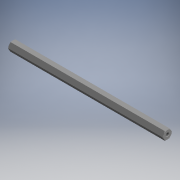
# Autodesk Inventor part: SLSBF7-130-M3-N3
Saved by Autodesk Inventor 2017.3 (Build 213256000, 256)
## iProperties
Part Number: SLSBF7-130-M3-N3
Material: Generic
Catalog Web Link: www.cadenas.de
Description: NLSBF, LSBF, PLSBF, BLSBF, SLSBF, ALSBF, ABLSBF-Hex Posts - Both Ends Tapped - L Dimension, Thread Dia. Configurable -
Vendor: MISUMI
Document SubType Name: Modeling
Designer: partserver
Manufacturer: MISUMI
Mass: 5.43424 g
Surface Area: 33.6052 cm^2
Volume: 5.43424 cm^3
Density: 1 g/cm^3
Appearance: PSOLRGB-175-175-175
Category: PARTsolutions
Company: MISUMI
Title: SLSBF7-130-M3-N3
Author: Cadenas PARTsolutions
Comments: Hex Posts - Both Ends Tapped - L Dimension, Thread Dia. Configurable -
PSOL_IDENT_0: {$CADENAS_DATA\23d-libs\misumi\metric\19_posts_stands\plsbf.prj},250 {VTYP=3D},{NB=SLSBF7-130-M3-N3}
PSOL_IDENT_1: ,{LINA=SLSBF7-130-M3-N3},{NN=NLSBF, LSBF, PLSBF, BLSBF, SLSBF, ALSBF, ABLSBF},{DATE=02.06.2021 23:49
PSOL_IDENT_2: :08},{GEOMDATE=25.03.2021 00:56:23},{VERSION=},{LINEID=50},{WBVAR=MAT,ST,M,N,ALT1,L,ALT4,ALT2,ALT3},
PSOL_IDENT_3: {WBNUMERIC=M,N,L}  {NB=SLSBF7-130-M3-N3},{LINA=SLSBF7-130-M3-N3},{KT=DUMMY},{PN=SLSBF7-130-M3-N3},{T
PSOL_IDENT_4: YPE=SLSBF},{MAT=304},{MATALG= 'LCS','Low Carbon Steel','304','SUS304','A2011','A2011 Aluminum Alloy'
PSOL_IDENT_5: },{ST=-},{STALG= '-','-' },{B=7},{M=3},{MALG=[3,4,5]},{N=3},{NALG=[3,4,5]},{ALT1=},{L=130.0},{LALG=
PSOL_IDENT_6: [15:200/0.5]},{LMIN=15},{LMIN1=12},{LMIN1ALG=12},{LMIN2=15.000},{C=8.1},{ALT4=},{ALT4ALG= '', 'w/o L
PSOL_IDENT_7: VC (L Dimension Accuracy Change)', 'LVC', 'with LVC (L Dimension Accuracy Change)'},{ALT4PN=},{ALT2=
PSOL_IDENT_8: },{ALT2ALG='','w/o MD (Left End Change The Effective Tap Depth)','MD','with MD (Left End Change The
PSOL_IDENT_9: Effective Tap Depth)'},{ALT2PN=},{ALT3=},{ALT3ALG='','w/o ND (Right End Change The Effective Tap Dep
PSOL_IDENT_10: th)','ND','with ND (Right End Change The Effective Tap Depth)'},{ALT3PN=},{MAV=3},{MPITCH=0.5},{NPIT
PSOL_IDENT_11: CH=0.5},{NDEPT=9},{MDEPT=9},{M3D=6},{N3D=6}
NB: SLSBF7-130-M3-N3
NN: NLSBF, LSBF, PLSBF, BLSBF, SLSBF, ALSBF, ABLSBF
NT: Hex Posts - Both Ends Tapped - L Dimension, Thread Dia. Configurable -
NBSYN: $PN.
LINA: SLSBF7-130-M3-N3
CATALOG: Misumi
PN: SLSBF7-130-M3-N3
MAT: SUS304
ST: -
B: 7
M: 3
N: 3
ALT1: w/o LKC (L Dimension Tolerance)
L: 130
C: 8.1
ALT4: w/o LVC (L Dimension Accuracy Change)
ALT2: w/o MD (Left End Change The Effective Tap Depth)
ALT3: w/o ND (Right End Change The Effective Tap Depth)
SUPPLIER: MISUMI
ARTICLENO: SLSBF7-130-M3-N3
BOMINFO: SLSBF7-130-M3-N3
CREATOR: CADENAS GmbH
Autodesk Inventor part; units mm, degrees
sketch "Sketch_1" plane through (0, 0, 0) normal (0, 0, 1) x (1, 0, 0)
  line L0 (130, 0) -> (0, 0)
  line L1 (0, 0) -> (0, 3.5)
  line L2 (0, 3.5) -> (0.6062, 4.55)
  line L3 (0.6062, 4.55) -> (129.3938, 4.55)
  line L4 (129.3938, 4.55) -> (130, 3.5)
  line L5 (130, 3.5) -> (130, 0)
  line L6 (130, 0) -> (0, 0)
  constraints: 14 end point
revolve "Revolution1" add sketch "Sketch_1" angle 360 about axis through (130, 0, 0) along (1, 0, 0)
sketch "Sketch_2" plane through (0, 0, 0) normal (1, 0, 0) x (0, 1, 0)
  line L0 (7, 7) -> (-7, 7)
  line L1 (-7, 7) -> (-7, -7)
  line L2 (-7, -7) -> (7, -7)
  line L3 (7, -7) -> (7, 7)
  line L4 (-2.0207, 3.5) -> (-4.0415, 0)
  line L5 (-4.0415, 0) -> (-2.0207, -3.5)
  line L6 (-2.0207, -3.5) -> (2.0207, -3.5)
  line L7 (2.0207, -3.5) -> (4.0415, 0)
  line L8 (4.0415, 0) -> (2.0207, 3.5)
  line L9 (2.0207, 3.5) -> (-2.0207, 3.5)
  constraints: 20 end point
extrude "Extrusion1" cut sketch "Sketch_2" along normal blind 130
sketch "Sketch3" plane through (0, 0, 0) normal (-1, 0, 0) x (0, 0, 1)
  point P0 (0, 0)
hole "Hole1" at (0, 0, 0) direction (1, 0, 0) diameter 2.459 depth 8.2901 tip angle 120 countersink diameter 3 countersink angle 90 thread size "M3x0.5" class "6H" standard "ISO Metric profile"
sketch "Sketch4" plane through (130, 0, 0) normal (1, 0, 0) x (0, 0, -1)
  point P0 (0, 0)
hole "Hole2" at (130, 0, 0) direction (-1, 0, 0) diameter 2.459 depth 8.2901 tip angle 120 countersink diameter 3 countersink angle 90 thread size "M3x0.5" class "6H" standard "ISO Metric profile"
ref_plane "C3_XY" through (130, 0, 0) normal (-1, 0, 0) x (0, 0, -1)
ref_plane "C3_YZ" through (130, 0, 0) normal (0, 0, -1) x (0, -1, 0)
ref_plane "C3_ZX" through (130, 0, 0) normal (0, -1, 0) x (-1, 0, 0)
body "Solid1"
